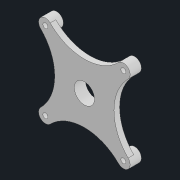
# Autodesk Inventor part: Part1
Saved by Autodesk Inventor 2022 (Build 260153000, 153)
## iProperties
Created: 2021-10-28
Part Number: Part1
Material: 一般
Document SubType Name: Modeling
Designer: Yuta Kage
Density: 1 g/cm^3
Appearance: 既定
Author: Yuta Kage
Autodesk Inventor part; units mm, degrees
ref_plane "YZ Plane" through (0, 0, 0) normal (1, 0, 0) x (0, 1, 0)
ref_plane "XZ Plane" through (0, 0, 0) normal (0, 1, 0) x (-1, 0, 0)
ref_plane "XY Plane" through (0, 0, 0) normal (0, 0, 1) x (1, 0, 0)
sketch "スケッチ1" plane through (0, 0, 0) normal (0, 0, 1) x (1, 0, 0)
  circle A0 centre (0, 0) radius 49 construction
  circle A1 centre (-34.6482, 34.6482) radius 6
  circle A2 centre (-34.6482, -34.6482) radius 6
  circle A3 centre (34.6482, -34.6482) radius 6
  circle A4 centre (34.6482, 34.6482) radius 6
  circle A5 centre (0, 69.2965) radius 43
  circle A6 centre (-69.2965, 0) radius 43
  circle A7 centre (0, -69.2965) radius 43
  circle A8 centre (69.2965, 0) radius 43
  line L0 (-40.6482, -40.6482) -> (40.6482, -40.6482)
  line L1 (40.6482, -40.6482) -> (40.6482, 40.6482)
  line L2 (40.6482, 40.6482) -> (-40.6482, 40.6482)
  line L3 (-40.6482, 40.6482) -> (-40.6482, -40.6482)
  line L4 (-40.6482, -40.6482) -> (40.6482, 40.6482) construction
  line L5 (40.6482, -40.6482) -> (-40.6482, 40.6482) construction
  line L6 (0, 69.2965) -> (-69.2965, 0)
  circle A9 centre (0, 0) radius 13
  point P0 (0, 26.2965)
  point P1 (-26.2965, 0)
  point P2 (0, -26.2965)
  point P3 (26.2965, 0)
  point P4 (38.8909, -30.4056)
  point P5 (38.8909, 30.4056)
  point P6 (30.4056, 38.8909)
  point P7 (-30.4056, 38.8909)
  point P8 (-38.8909, 30.4056)
  point P9 (-38.8909, -30.4056)
  point P10 (-30.4056, -38.8909)
  point P11 (30.4056, -38.8909)
  dimension "d0" = 98
  dimension "d1" = 12
  dimension "d4" = 360
  dimension "d9" = 360
  dimension "d27" = 26
  constraints: 14 end point, 5 centre point, 3 midpoint, 2 coincident, 2 parallel, 2 tangent, 1 horizontal, 1 horizontal alignment, 1 perpendicular, 1 vertical alignment, 39 other
  measures "d1" diameter of A1
  measures "d27" diameter of A9
extrude "押し出し1" add sketch "スケッチ1" along normal blind 5 contours A1 L6 | A1 A5 A4 A8 A3 A7 A2 A6 | L6 A1 | A4 | A2 | A3 | A9
extrude "押し出し4" add sketch "スケッチ1" against normal blind 5 contours A1 L6 | L6 A1 | A4 | A2 | A3 | A9
sketch "スケッチ5" plane through (0, 0, -5) normal (0, 0, -1) x (-1, 0, 0)
  circle A0 centre (0, 0) radius 9
  dimension "d28" = 18
  constraints: 1 centre point, 1 coincident
  measures "d28" diameter of A0
extrude "押し出し5" cut sketch "スケッチ5" against normal through all
sketch "スケッチ6" plane through (-34.6482, -34.6482, -5) normal (0, 0, -1) x (-1, 0, 0)
  circle A0 centre (-34.6482, 34.6482) radius 9 projected
  circle A1 centre (-34.6482, 34.6482) radius 13 projected
  circle A2 centre (-69.2965, 0) radius 6 projected
  circle A3 centre (0, 0) radius 6 projected
  circle A4 centre (0, 69.2965) radius 6 projected
  circle A5 centre (-69.2965, 69.2965) radius 6 projected
hole "穴1" at (-34.6482, -34.6482, -5) at (34.6482, -34.6482, -5) at (-34.6482, 34.6482, -5) at (34.6482, 34.6482, -5) direction (0, 0, 1) diameter 4.5 end through all clearance for "Flat Head Machine Screw" size "M4" standard "Ansi Metric M Profile"
